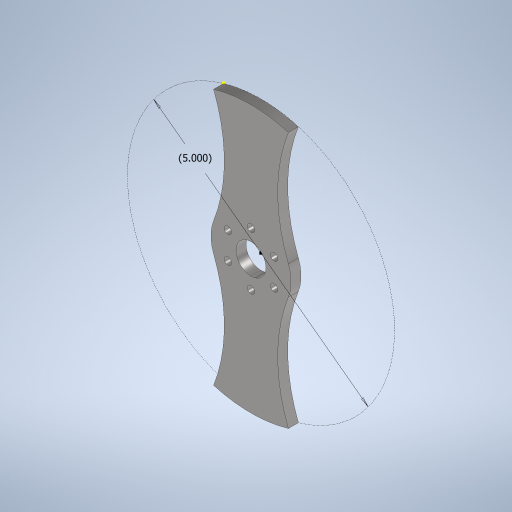
# Autodesk Inventor part: Blade (Bar)
Saved by Autodesk Inventor 2023.2 (Build 272271000, 271)
## iProperties
Created: 2022-06-12
Part Number: Blade (Bar)
Material: Stainless Steel
Document SubType Name: Modeling
Designer: Nathan Cai
Density: 8 g/cm^3
Appearance: Semi-Polished
Mass: 209.485 g
Surface Area: 133.7 cm^2
Volume: 26.1856 cm^3
Author: Nathan Cai
Autodesk Inventor part; units mm, degrees
ref_plane "YZ Plane" through (0, 0, 0) normal (1, 0, 0) x (0, 1, 0)
ref_plane "XZ Plane" through (0, 0, 0) normal (0, 1, 0) x (-1, 0, 0)
ref_plane "XY Plane" through (0, 0, 0) normal (0, 0, 1) x (1, 0, 0)
sketch "Sketch1" plane through (0, 0, 0) normal (0, 0, 1) x (1, 0, 0)
  circle A0 centre (0, 0) radius 7.1437
  line L0 (0, 0) -> (0, 12.7) construction
  circle A1 centre (0, 12.7) radius 1.7526
  circle A2 centre (-10.9985, 6.35) radius 1.7526
  circle A3 centre (-10.9985, -6.35) radius 1.7526
  circle A4 centre (0, -12.7) radius 1.7526
  circle A5 centre (10.9985, -6.35) radius 1.7526
  circle A6 centre (10.9985, 6.35) radius 1.7526
  circle A7 centre (0, 0) radius 63.5 construction
  line L1 (-12.7, -62.217) -> (12.7, -62.217) construction
  line L2 (12.7, -62.217) -> (12.7, 62.217) construction
  line L3 (12.7, 62.217) -> (-12.7, 62.217) construction
  line L4 (-12.7, 62.217) -> (-12.7, -62.217) construction
  line L5 (-12.7, -62.217) -> (12.7, 62.217) construction
  line L6 (12.7, -62.217) -> (-12.7, 62.217) construction
  line L7 (0, 63.5) -> (0, -63.5) construction
  line L8 (0, 0) -> (17.778, 60.9606) construction
  circle A8 centre (0, 0) radius 53.975 construction
  circle A9 centre (0, 0) radius 19.05
  line L9 (17.778, 60.9606) -> (14.309, 52.0438) construction
  arc A10 (17.778, 60.9606) -> (-17.778, 60.9606) centre (0, 0) ccw
  line L10 (-12.7, 0) -> (12.7, 0) construction
  arc A11 (-17.778, -60.9606) -> (17.778, -60.9606) centre (0, 0) ccw
  arc A12 (17.778, 60.9606) -> (17.7587, 6.8943) centre (87.3276, 33.9025) ccw
  arc A13 (-17.7587, 6.8943) -> (-17.778, 60.9606) centre (-87.3276, 33.9025) ccw
  arc A14 (17.7587, -6.8943) -> (17.778, -60.9606) centre (87.3276, -33.9025) ccw
  arc A15 (-17.778, -60.9606) -> (-17.7587, -6.8943) centre (-87.3276, -33.9025) ccw
  point P0 (0, 62.217)
  point P1 (0, -53.975)
  point P2 (17.7587, -6.8943)
  point P3 (-17.7587, -6.8943)
  point P4 (-17.7587, 6.8943)
  dimension "d10" = 38.1
  dimension "d0" = 14.2875
  dimension "d1" = 12.7
  dimension "d2" = 3.5052
  dimension "d5" = 360
  dimension "d7" = 127
  dimension "d8" = 25.4
  dimension "d9" = 9.525
  dimension "d11" = 5
  constraints: 22 end point, 19 point on circle, 15 centre point, 9 symmetric about line, 7 midpoint, 4 coincident, 2 parallel, 2 perpendicular, 2 tangent, 1 horizontal, 1 point on line, 1 vertical, 22 other
  measures "d0" diameter of A0
  measures "d1" distance of L0.start L0.end
  measures "d2" diameter of A1
  measures "d7" diameter of A7
  measures "d8" distance of L3.end L2.end
  measures "d9" radial gap between concentric circles of A7 A8
  measures "d11" angle of L9 L8
extrude "Extrusion1" add sketch "Sketch1" along normal blind 4.7625
sketch "Sketch3" plane through (0, 0, 0) normal (0, 0, -1) x (-1, 0, 0)
  circle A0 centre (0, 0) radius 63.5 construction
  point P0 (17.778, 60.9606)
  dimension "d25" = 127
  constraints: 1 coincident, 3 other
body "Solid1"
